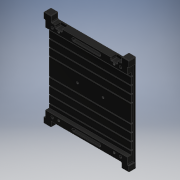
# Autodesk Inventor part: -Y
Saved by Autodesk Inventor 2018 (Build 220112000, 112)
## iProperties
Created: 2018-07-04
Part Number: -Y
Material: Aluminum 6061
Document SubType Name: Modeling
Designer: Bradley
Density: 2.7 g/cm^3
Appearance: Anodized - Dark Gray
Mass: 115.313 g
Surface Area: 282.648 cm^2
Volume: 42.7085 cm^3
Author: Bradley
Autodesk Inventor part; units mm, degrees
ref_plane "YZ Plane" through (0, 0, 0) normal (1, 0, 0) x (0, 1, 0)
ref_plane "XZ Plane" through (0, 0, 0) normal (0, 1, 0) x (-1, 0, 0)
ref_plane "XY Plane" through (0, 0, 0) normal (0, 0, 1) x (1, 0, 0)
sketch "Sketch1" plane through (0, 0, 0) normal (0, 1, 0) x (-1, 0, 0)
  line L0 (50, 57) -> (50, -56.5)
  line L1 (50, -56.5) -> (41.5, -56.5)
  line L2 (41.5, -56.5) -> (41.5, -50)
  line L3 (41.5, -50) -> (-41.5, -50)
  line L4 (-41.5, -50) -> (-41.5, -56.5)
  line L5 (-41.5, -56.5) -> (-50, -56.5)
  line L6 (-50, -56.5) -> (-50, 57)
  line L7 (-50, 57) -> (-41.5, 57)
  line L8 (-41.5, 57) -> (-41.5, 50)
  line L9 (-41.5, 50) -> (41.5, 50)
  line L10 (41.5, 50) -> (41.5, 57)
  line L11 (50, 57) -> (41.5, 57)
  point P0 (0, 0)
  point P1 (0, 0)
  point P2 (0, 50)
  dimension "d0" = 100
  dimension "d1" = 8.5
  dimension "d2" = 113.5
  dimension "d3" = 7
  dimension "d4" = 6.5
  dimension "d5" = 56.5
  constraints: 24 end point, 8 perpendicular, 7 point on line, 1 coincident, 1 collinear, 1 midpoint, 1 vertical, 1 vertical alignment
  measures "d0" distance between parallel lines of L6 L0
  measures "d1" distance of L0.start L10.end
  measures "d2" distance of L0.start L0.end
  measures "d3" distance of L9.end L10.end
  measures "d4" distance of L1.end L2.end
  measures "d5" distance from line of point (0, 0) L1
extrude "Extrusion1" add sketch "Sketch1" along normal mid plane 8.5
sketch "Sketch2" plane through (50, -4.25, -56.5) normal (1, 0, 0) x (0, 0, -1)
  line L0 (0, 8.5) -> (0, 0) projected
  line L1 (-113.5, 8.5) -> (0, 8.5) projected
  line L2 (-113.5, 8.5) -> (-113.5, 0) projected
  line L3 (0, 0) -> (-113.5, 0) projected
  line L4 (-106.5, 8.5) -> (-106.5, 0) projected
  line L5 (-6.5, 8.5) -> (-6.5, 0) projected
  line L6 (0, 0) -> (-113.5, 0) projected
  line L7 (-98.5, 0) -> (-98.5, 4.5)
  line L8 (-98.5, 4.5) -> (-14.5, 4.5)
  line L9 (-14.5, 4.5) -> (-14.5, 0)
  line L10 (-46.55, 4.5) -> (-45.45, 4.5)
  line L11 (-45.45, 4.5) -> (-45.45, 6.5)
  line L12 (-45.45, 6.5) -> (-46.55, 6.5)
  line L13 (-46.55, 6.5) -> (-46.55, 4.5)
  line L14 (0, 8.5) -> (-113.5, 8.5) construction
  line L15 (-56.5, 8.5) -> (-56.5, 0) construction
  line L16 (-36.45, 4.5) -> (-36.45, 6.5)
  line L17 (-37.55, 4.5) -> (-36.45, 4.5)
  line L18 (-37.55, 6.5) -> (-37.55, 4.5)
  line L19 (-36.45, 6.5) -> (-37.55, 6.5)
  line L20 (-27.45, 4.5) -> (-27.45, 6.5)
  line L21 (-28.55, 4.5) -> (-27.45, 4.5)
  line L22 (-28.55, 6.5) -> (-28.55, 4.5)
  line L23 (-27.45, 6.5) -> (-28.55, 6.5)
  line L24 (-18.45, 4.5) -> (-18.45, 6.5)
  line L25 (-19.55, 4.5) -> (-18.45, 4.5)
  line L26 (-19.55, 6.5) -> (-19.55, 4.5)
  line L27 (-18.45, 6.5) -> (-19.55, 6.5)
  line L28 (-66.45, 4.5) -> (-67.55, 4.5)
  line L29 (-67.55, 4.5) -> (-67.55, 6.5)
  line L30 (-67.55, 6.5) -> (-66.45, 6.5)
  line L31 (-66.45, 6.5) -> (-66.45, 4.5)
  line L32 (-76.55, 4.5) -> (-76.55, 6.5)
  line L33 (-75.45, 4.5) -> (-76.55, 4.5)
  line L34 (-75.45, 6.5) -> (-75.45, 4.5)
  line L35 (-76.55, 6.5) -> (-75.45, 6.5)
  line L36 (-85.55, 4.5) -> (-85.55, 6.5)
  line L37 (-84.45, 4.5) -> (-85.55, 4.5)
  line L38 (-84.45, 6.5) -> (-84.45, 4.5)
  line L39 (-85.55, 6.5) -> (-84.45, 6.5)
  line L40 (-94.55, 4.5) -> (-94.55, 6.5)
  line L41 (-93.45, 4.5) -> (-94.55, 4.5)
  line L42 (-93.45, 6.5) -> (-93.45, 4.5)
  line L43 (-94.55, 6.5) -> (-93.45, 6.5)
  point P0 (-56.5, 4.25)
  point P1 (-56.5, 4.25)
  point P2 (-46, 6.5)
  point P3 (-37, 6.5)
  point P4 (-28, 6.5)
  point P5 (-19, 6.5)
  point P6 (-67, 6.5)
  point P7 (-76, 6.5)
  point P8 (-85, 6.5)
  point P9 (-94, 6.5)
  dimension "d8" = 4
  dimension "d9" = 8
  dimension "d10" = 8
  dimension "d11" = 1.1
  dimension "d14" = 9
  dimension "d19" = 21
  dimension "d20" = 2
  constraints: 72 end point, 20 symmetric about line, 5 point on line, 4 perpendicular, 3 parallel, 2 horizontal, 2 midpoint, 1 coincident, 27 other
  measures "d8" distance between parallel lines of L1 L8
  measures "d9" distance between parallel lines of L7 L4
  measures "d10" distance between parallel lines of L5 L9
  measures "d11" distance of L11.end L12.end
  measures "d14" distance of L11.end L16.end
  measures "d19" distance of point (-46, 6.5) point (-67, 6.5)
  measures "d20" distance between parallel lines of L1 L12
extrude "Extrusion2" cut sketch "Sketch2" against normal through all contours L3 L7 L8 L9 | L8 L26 L27 L24 | L40 L43 L42 L8 | L8 L22 L23 L20 | L36 L39 L38 L8 | L8 L18 L19 L16 | L32 L35 L34 L8 | L8 L13 L12 L11 | L29 L30 L31 L8
fillet "Fillet1" radius 1 6 edges at (41.5, 0, 50) (-41.5, 0, 50) (-41.5, 0, -50) (41.5, 0, -50) (50, 4.25, 0.25) (-50, 4.25, 0.25)
chamfer "Chamfer1" distance 0.5 angle 45 30 edges at (45.75, -4.25, 57) (41.5, 0, 57) (49.7071, 3.9571, 57) (50, -0.5, 57) (45.25, 4.25, 57) (-45.25, 4.25, 57) (-49.7071, 3.9571, 57) (-50, -0.5, 57) (-41.5, 0, 57) (-45.75, -4.25, 57) (-41.5, 0, -56.5) (-45.75, -4.25, -56.5) (-45.25, 4.25, -56.5) (-49.7071, 3.9571, -56.5) (-50, -0.5, -56.5) (50, -0.5, -56.5) (49.7071, 3.9571, -56.5) (45.25, 4.25, -56.5) (41.5, 0, -56.5) (45.75, -4.25, -56.5) (0, 4.25, -50) (-41.2071, 4.25, -50.2929) (-41.5, 4.25, -53.75) (41.2071, 4.25, -50.2929) (41.5, 4.25, -53.75) (0, 4.25, 50) (41.2071, 4.25, 50.2929) (41.5, 4.25, 54) (-41.2071, 4.25, 50.2929) (-41.5, 4.25, 54)
sketch "Sketch3" plane through (0, 4.25, 0) normal (0, 1, 0) x (1, 0, 0)
  line L0 (-32.5, 45) -> (32.5, 45) construction
  line L1 (32.5, 45) -> (32.5, -45) construction
  line L2 (32.5, -45) -> (-32.5, -45) construction
  line L3 (-32.5, -45) -> (-32.5, 45) construction
  line L4 (-32.5, 45) -> (32.5, -45) construction
  line L5 (32.5, 45) -> (-32.5, -45) construction
  line L6 (15, 0) -> (-15, 0) construction
  point P0 (0, 0)
  point P1 (0, 0)
  dimension "d27" = 30
  dimension "d28" = 65
  dimension "d29" = 90
  constraints: 14 end point, 6 coincident, 4 midpoint, 2 horizontal, 2 parallel, 1 perpendicular
  measures "d27" distance of L6.start L6.end
  measures "d28" distance of L1.end L2.end
  measures "d29" distance of L0.end L1.end
hole "Hole1" at (32.5, 4.25, 45) at (-32.5, 4.25, 45) at (-15, 4.25, 0) at (15, 4.25, 0) at (32.5, 4.25, -45) at (-32.5, 4.25, -45) direction (0, -1, 0) diameter 2.621 end through all thread size "M3x0.35" class "6H" standard "ANSI Metric M Profile"
sketch "Sketch4" plane through (0, -4.25, 0) normal (0, -1, 0) x (1, 0, 0)
  circle A0 centre (32.5, 45) radius 1.3105 projected
  line L0 (-50, 42) -> (50, 42) projected
  line L1 (50, 42) -> (50, 56.5) projected
  line L2 (41.5, 56.5) -> (50, 56.5) projected
  line L3 (-50, 56.5) -> (-41.5, 56.5) projected
  line L4 (-50, 56.5) -> (-50, 42) projected
  circle A1 centre (-32.5, 45) radius 1.3105 projected
  line L5 (0, 50) -> (0, 42) construction
  line L6 (50, 42) -> (-50, 42) construction
  line L7 (-36.55, 50) -> (-28.45, 50)
  line L8 (-28.45, 50) -> (-28.45, 46.95)
  line L9 (-28.45, 46.95) -> (-36.55, 46.95)
  line L10 (-36.55, 46.95) -> (-36.55, 50)
  line L11 (28.45, 50) -> (36.55, 50)
  line L12 (36.55, 50) -> (36.55, 46.95)
  line L13 (36.55, 46.95) -> (28.45, 46.95)
  line L14 (28.45, 46.95) -> (28.45, 50)
  line L15 (-15, 46) -> (15, 46) construction
  line L16 (-15, 44.45) -> (15, 44.45)
  line L17 (15, 47.55) -> (-15, 47.55)
  arc A2 (-15, 47.55) -> (-15, 44.45) centre (-15, 46) ccw
  arc A3 (15, 44.45) -> (15, 47.55) centre (15, 46) ccw
  line L18 (41.5, 56.5) -> (41.5, 51) projected
  arc A4 (40.5, 50) -> (41.5, 51) centre (40.5, 51) ccw projected
  line L19 (40.5, 50) -> (-40.5, 50) projected
  arc A5 (-41.5, 51) -> (-40.5, 50) centre (-40.5, 51) ccw projected
  line L20 (-41.5, 51) -> (-41.5, 56.5) projected
  point P0 (0, 0)
  point P1 (31.653, 44)
  point P2 (-31.653, 44)
  point P3 (0, 46)
  point P4 (-32.5, 46.95)
  dimension "d38" = 3.1
  dimension "d39" = 30
  dimension "d40" = 8.1
  dimension "d41" = 3.05
  constraints: 26 end point, 5 midpoint, 5 parallel, 4 point on circle, 4 tangent, 3 perpendicular, 2 centre point, 2 horizontal, 2 point on line, 1 collinear, 1 vertical alignment, 4 other
  measures "d38" distance between parallel lines of L16 L17
  measures "d39" distance of L17.start L17.end
  measures "d40" distance of L8.end L9.end
  measures "d41" distance of L9.end L7.start
extrude "Extrusion3" cut sketch "Sketch4" against normal blind 3.1 contours A2 L17 A3 L16
extrude "Extrusion4" cut sketch "Sketch4" against normal blind 6.6 contours L7 L8 L9 L10 | L12 L13 L14 L11
sketch "Sketch5" plane through (0, 4.25, 0) normal (0, 1, 0) x (1, 0, 0)
  circle A0 centre (32.5, 45) radius 1.3105 projected
  circle A1 centre (-15, 0) radius 1.3105 projected
  circle A2 centre (32.5, -45) radius 1.3105 projected
  circle A3 centre (-32.5, -45) radius 1.3105 projected
  circle A4 centre (15, 0) radius 1.3105 projected
  circle A5 centre (-32.5, 45) radius 1.3105 projected
  line L0 (-49, 56) -> (-42, 56) projected
  line L1 (-49, -56.5) -> (-49, 56) projected
  line L2 (-42, -56.5) -> (-49, -56.5) projected
  line L3 (-42, -51) -> (-42, -56.5) projected
  arc A6 (-40.5, -49.5) -> (-42, -51) centre (-40.5, -51) ccw projected
  line L4 (40.5, -49.5) -> (-40.5, -49.5) projected
  arc A7 (42, -51) -> (40.5, -49.5) centre (40.5, -51) ccw projected
  line L5 (42, -56.5) -> (42, -51) projected
  line L6 (49, -56.5) -> (42, -56.5) projected
  line L7 (49, 56) -> (49, -56.5) projected
  line L8 (42, 56) -> (49, 56) projected
  line L9 (42, 51) -> (42, 56) projected
  arc A8 (40.5, 49.5) -> (42, 51) centre (40.5, 51) ccw projected
  line L10 (-40.5, 49.5) -> (40.5, 49.5) projected
  arc A9 (-42, 51) -> (-40.5, 49.5) centre (-40.5, 51) ccw projected
  line L11 (-42, 56) -> (-42, 51) projected
  line L12 (40, -45.5) -> (-40, -45.5) construction
  line L13 (-40.5, -50) -> (40.5, -50) projected
  point P0 (0, 0)
  point P1 (0, -45.5)
  dimension "d50" = 80
  dimension "d51" = 4.5
  constraints: 2 coincident, 2 end point, 1 horizontal, 1 midpoint, 1 vertical alignment
  measures "d50" distance of L12.start L12.end
  measures "d51" distance between parallel lines of L13 L12
hole "Hole2" at (40, 4.25, 45.5) at (-40, 4.25, 45.5) direction (0, -1, 0) diameter 3.2 end through all counterbore diameter 6 counterbore depth 2.1 clearance for "Socket Head Cap Screw" size "M3" standard "Ansi Metric M Profile"
mirror "Mirror1" about plane through (0, 0, 0) normal (0, 0, 1) of "Hole2", "Extrusion3"
fillet "Fillet3" radius 1 4 edges at (-28.45, -0.95, 46.95) (-36.55, -0.95, 46.95) (36.55, -0.95, 46.95) (28.45, -0.95, 46.95)
chamfer "Chamfer3" distance 0.5 angle 45 22 edges at (32.5, -4.25, 46.95) (28.7429, -4.25, 47.2429) (28.45, -4.25, 48.975) (36.2571, -4.25, 47.2429) (36.55, -4.25, 48.975) (16.55, -4.25, 46) (0, -4.25, 44.45) (-16.55, -4.25, 46) (0, -4.25, 47.55) (16.55, -4.25, -46) (0, -4.25, -47.55) (-16.55, -4.25, -46) (0, -4.25, -44.45) (-28.45, -4.25, 48.975) (-28.7429, -4.25, 47.2429) (-32.5, -4.25, 46.95) (-36.2571, -4.25, 47.2429) (-36.55, -4.25, 48.975) (40, 4.25, 42.5) (-40, 4.25, 42.5) (-40, 4.25, -42.5) (40, 4.25, -42.5)
sketch "Sketch6" plane through (50, -4.25, 42) normal (1, 0, 0) x (0, 0, -1)
  line L0 (98, 7.5) -> (98, 0) projected
  line L1 (-14.5, 7.5) -> (98, 7.5) projected
  line L2 (-14.5, 0) -> (-14.5, 7.5) projected
  line L3 (0, 0) -> (-14.5, 0) projected
  line L4 (0, 0) -> (0, 4.5) projected
  line L5 (0, 4.5) -> (3.95, 4.5) projected
  line L6 (3.95, 4.5) -> (3.95, 6.5) projected
  line L7 (3.95, 6.5) -> (5.05, 6.5) projected
  line L8 (5.05, 6.5) -> (5.05, 4.5) projected
  line L9 (5.05, 4.5) -> (12.95, 4.5) projected
  line L10 (12.95, 4.5) -> (12.95, 6.5) projected
  line L11 (12.95, 6.5) -> (14.05, 6.5) projected
  line L12 (14.05, 6.5) -> (14.05, 4.5) projected
  line L13 (14.05, 4.5) -> (21.95, 4.5) projected
  line L14 (21.95, 4.5) -> (21.95, 6.5) projected
  line L15 (21.95, 6.5) -> (23.05, 6.5) projected
  line L16 (23.05, 6.5) -> (23.05, 4.5) projected
  line L17 (23.05, 4.5) -> (30.95, 4.5) projected
  line L18 (30.95, 4.5) -> (30.95, 6.5) projected
  line L19 (30.95, 6.5) -> (32.05, 6.5) projected
  line L20 (32.05, 6.5) -> (32.05, 4.5) projected
  line L21 (32.05, 4.5) -> (51.95, 4.5) projected
  line L22 (51.95, 4.5) -> (51.95, 6.5) projected
  line L23 (51.95, 6.5) -> (53.05, 6.5) projected
  line L24 (53.05, 6.5) -> (53.05, 4.5) projected
  line L25 (53.05, 4.5) -> (60.95, 4.5) projected
  line L26 (60.95, 4.5) -> (60.95, 6.5) projected
  line L27 (60.95, 6.5) -> (62.05, 6.5) projected
  line L28 (62.05, 6.5) -> (62.05, 4.5) projected
  line L29 (62.05, 4.5) -> (69.95, 4.5) projected
  line L30 (69.95, 4.5) -> (69.95, 6.5) projected
  line L31 (69.95, 6.5) -> (71.05, 6.5) projected
  line L32 (71.05, 6.5) -> (71.05, 4.5) projected
  line L33 (71.05, 4.5) -> (78.95, 4.5) projected
  line L34 (78.95, 4.5) -> (78.95, 6.5) projected
  line L35 (78.95, 6.5) -> (80.05, 6.5) projected
  line L36 (80.05, 6.5) -> (80.05, 4.5) projected
  line L37 (80.05, 4.5) -> (84, 4.5) projected
  line L38 (84, 4.5) -> (84, 0) projected
  line L39 (98, 0) -> (84, 0) projected
  line L40 (-14.5, 0) -> (0, 0) projected
  line L41 (-8.05, 0) -> (-8.05, 7.05)
  line L42 (-8.05, 7.05) -> (92.05, 7.05)
  line L43 (92.05, 7.05) -> (92.05, 0)
  line L44 (98, 0) -> (84, 0) projected
  line L45 (-14.5, -41.5) -> (98, -41.5) construction
  line L46 (98, 8.5) -> (-14.5, 8.5) projected
  point P0 (42, 4.25)
  point P1 (42, 7.05)
  dimension "d63" = 100.1
  dimension "d64" = 50
  dimension "d65" = 97.1
  constraints: 8 end point, 3 vertical alignment, 2 parallel, 2 point on line, 1 horizontal, 1 midpoint, 1 perpendicular
  measures "d63" distance of L41.end L42.end
  measures "d64" distance between parallel lines of L45 L46
  measures "d65" diameter of L42 L45
extrude "Extrusion5" cut sketch "Sketch6" against normal blind 2 contours L39 L38 L37 L36 L35 L34 L33 L32 L31 L30 L29 L28 L27 L26 L25 L24 L23 L22 L21 L20 L19 L18 L17 L16 L15 L14 L13 L12 L11 L10 L9 L8 L7 L6 L5 L4 L3 L41 L42 L43
mirror "Mirror2" about plane through (0, 0, 0) normal (1, 0, 0) of "Extrusion5"
fillet "Fillet4" radius 1 4 edges at (48, -0.725, 50.05) (48, -0.725, -50.05) (-48, -0.725, -50.05) (-48, -0.725, 50.05)
sketch "Sketch7" plane through (-42, -3.75, -56.5) normal (0, 0, -1) x (-1, 0, 0)
  line L0 (0, 0) -> (0, 7.5) projected
  line L1 (7.5, 0) -> (0, 0) projected
  line L2 (7.5, 7) -> (7.5, 0) projected
  arc A0 (7.5, 7) -> (7, 7.5) centre (7, 7) ccw projected
  line L3 (0, 7.5) -> (7, 7.5) projected
  point P0 (-42, 3.75)
  point P1 (3.75, 3.75)
  point P2 (3.75, 0)
  point P3 (0, 3.75)
  constraints: 2 midpoint, 1 horizontal alignment, 1 vertical alignment
hole "Hole3" at (-45.75, 0, -56.5) direction (0, 0, 1) diameter 3.404 depth 11.5 tip angle 118 thread size "8-36 UNF" class "2B" standard "ANSI Unified Screw Threads"
body "Solid1"
